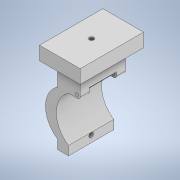
# Autodesk Inventor part: Part1
Saved by Autodesk Inventor 2021 (Build 250183000, 183)
## iProperties
Created: 2021-05-12
Part Number: Part1
Material: Generic
Document SubType Name: Modeling
Designer: chick
Density: 1 g/cm^3
Appearance: Default
Author: chick
Autodesk Inventor part; units mm, degrees
ref_plane "YZ Plane" through (0, 0, 0) normal (1, 0, 0) x (0, 1, 0)
ref_plane "XZ Plane" through (0, 0, 0) normal (0, 1, 0) x (-1, 0, 0)
ref_plane "XY Plane" through (0, 0, 0) normal (0, 0, 1) x (1, 0, 0)
sketch "Sketch2" plane through (0, 0, 0) normal (0, 0, 1) x (1, 0, 0)
  line L0 (0, 50) -> (0, 0)
  line L1 (0, 0) -> (50, 0)
  line L2 (50, 0) -> (50, 50)
  line L3 (50, 50) -> (0, 50)
  dimension "base" = 50
  dimension "d1" = 50
  constraints: 8 end point, 3 perpendicular, 1 vertical
  measures "base" distance of L1.end L2.end
  measures "d1" distance of L2.end L0.start
extrude "Extrusion1" add sketch "Sketch2" along normal mid plane 100
sketch "Sketch12" plane through (0, 0, 50) normal (0, 0, 1) x (1, 0, 0)
  line L0 (0, -120) -> (24, -120)
  line L1 (0, -120) -> (0, -100)
  line L2 (0, 0) -> (50, 0) projected
  arc A0 (0, 0) -> (0, -100) centre (33.1662, -50) ccw
  arc A1 (24, 0) -> (24, -100) centre (57.1662, -50) ccw
  line L3 (24, -100) -> (24, -120)
  point P0 (24.2536, -50)
  dimension "d56" = 100
  dimension "d57" = 50
  dimension "d58" = 60
  dimension "d59" = 20
  dimension "d61" = 24
  dimension "d103" = 60
  dimension "d110" = 24
  dimension "d111" = 20
  constraints: 6 end point, 4 point on circle, 2 centre point, 2 vertical, 1 horizontal, 1 point on line
  measures "d56" distance of L1.end L2.start
  measures "d57" distance from line of point (24.254, -50) L2
  measures "d58" radius of A0
  measures "d59" distance of L0.start L1.end
  measures "d61" distance of A1.start L2.start
  measures "d103" radius of A1
  measures "d110" distance of L0.start L0.end
  measures "d111" distance of L3.start L0.end
extrude "Extrusion6" add sketch "Sketch12" against normal blind 100
sketch "Sketch13" plane through (0, 50, 50) normal (0, 1, 0) x (1, 0, 0)
  line L0 (50, 100) -> (50, 0) projected
  line L1 (0, 100) -> (50, 100) projected
  line L2 (-20, 120) -> (70, 120)
  line L3 (70, 120) -> (70, -20)
  line L4 (70, -20) -> (-20, -20)
  line L5 (-20, -20) -> (-20, 120)
  line L6 (-20, 120) -> (70, -20) construction
  line L7 (70, 120) -> (-20, -20) construction
  point P0 (0, 50)
  point P1 (25, 50)
  dimension "d68" = 25
  dimension "d69" = 50
  dimension "d70" = 140
  dimension "d71" = 90
  constraints: 12 end point, 2 midpoint, 2 parallel, 1 horizontal, 1 perpendicular
  measures "d68" distance from line of L0 point (25, 50)
  measures "d69" distance from line of L1 point (25, 50)
  measures "d70" distance of L2.end L3.end
  measures "d71" distance of L3.end L4.end
extrude "Extrusion7" add sketch "Sketch13" along normal blind 30
sketch "Sketch16" plane through (0, 80, 50) normal (0, 1, 0) x (1, 0, 0)
  circle A0 centre (25, 50) radius 5
  point P0 (0, 50)
  dimension "d74" = 10
  constraints: 1 centre point, 1 coincident
  measures "d74" diameter of A0
hole "Hole3" at (25, 80, 0) direction (0, -1, 0) diameter 8 depth 80 tip angle 118 counterbore diameter 10 counterbore depth 3
sketch "Sketch17" plane through (0, 0, 50) normal (0, 0, 1) x (1, 0, 0)
  line L0 (50, 0) -> (50, 50) projected
  line L1 (24, 0) -> (50, 0) projected
  circle A0 centre (43, 7) radius 3.5
  point P0 (0, 0)
  point P1 (10, 0)
  point P2 (43, 10.5)
  dimension "d84" = 7
  dimension "d82" = 7
  dimension "d83" = 7
  constraints: 1 coincident, 1 vertical alignment, 2 other
  measures "d82" distance from line of L0 point (43, 7)
  measures "d83" distance from line of L1 point (43, 7)
extrude "Extrusion8" cut sketch "Sketch17" against normal blind 100
sketch "Sketch18" plane through (50, 0, 50) normal (1, 0, 0) x (0, 0, -1)
  line L0 (0, 0) -> (100, 0) projected
  line L1 (20, 0) -> (80, 0)
  line L2 (0, 0) -> (0, 50) projected
  line L3 (20, 0) -> (20, 14)
  line L4 (20, 14) -> (80, 14)
  line L5 (0, 10.5) -> (100, 10.5) projected
  line L6 (80, 14) -> (80, 0)
  line L7 (100, 50) -> (100, 0) projected
  point P0 (50, 0)
  point P1 (80, 10.5)
  point P2 (20, 10.5)
  dimension "d104" = 14
  dimension "d108" = 20
  dimension "d109" = 20
  constraints: 8 end point, 2 point on line, 1 collinear, 1 parallel, 1 perpendicular, 1 vertical
  measures "d104" distance of L1.start L3.end
  measures "d108" distance between parallel lines of L2 L3
  measures "d109" distance between parallel lines of L7 L6
extrude "Extrusion9" cut sketch "Sketch18" against normal blind 13 contours L3 L5 L6 L0 | L3 L4 L6 L5
sketch "Sketch19" plane through (0, -120, 50) normal (-1, 0, 0) x (0, 0, 1)
  line L0 (0, 0) -> (-100, 0) projected
  circle A0 centre (-50, 15) radius 5
  point P0 (-50, 120)
  dimension "d91" = 15
  dimension "d92" = 10
  constraints: 1 centre point, 1 coincident
  measures "d91" distance from line of L0 point (-50, 15)
  measures "d92" diameter of A0
hole "Hole4" at (0, -105, 0) direction (1, 0, 0) diameter 10 end through all
fillet "Fillet1" radius 6 2 edges at (50, 0, 40) (50, 0, -40)
equation "\"d1\" = base"
equation "\"d56\" = arm_vertical_length"
equation "\"d59\" = connection_length"
equation "\"d61\" = arm_thickness"
equation "\"d103\" = d58"
equation "\"d110\" = d61"
equation "\"d111\" = connection_length"
equation "\"d70\" = platform_length"
equation "\"d71\" = platform_width"
equation "\"d74\" = cover_mountHole_diameter"
equation "\"d109\" = d108"
equation "\"arm_thickness\" = 24"
equation "\"arm_vertical_length\" = 100"
equation "\"connection_length\" = 20"
equation "\"platform_length\" = 140"
equation "\"platform_width\" = 90"
equation "\"cover_mountHole_diameter\" = 10"
body "Solid1"
